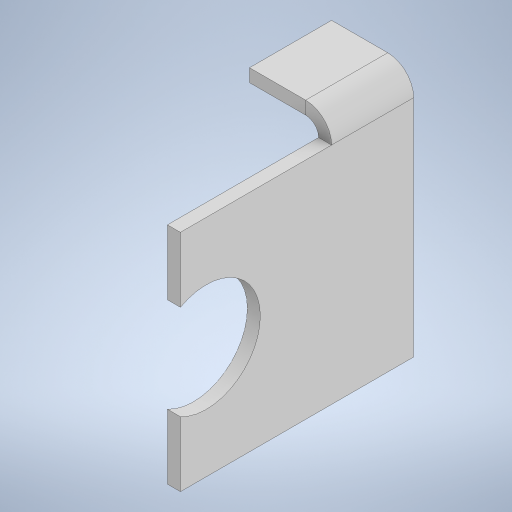
# Autodesk Inventor part: hipjoint_toleg_under_down_right
Saved by Autodesk Inventor 2024.1 (Build 281209000, 209)
## iProperties
Created: 2024-10-09
Part Number: hipjoint_toleg_under_down_right
Material: 一般
Document SubType Name: Sheet Metal
Designer: hibik
Density: 1 g/cm^3
Sheet Metal Rule: Default_mm
Appearance: 既定
Author: hibik
Autodesk Inventor part; units mm, degrees
ref_plane "YZ Plane" through (0, 0, 0) normal (1, 0, 0) x (0, 1, 0)
ref_plane "XZ Plane" through (0, 0, 0) normal (0, 1, 0) x (-1, 0, 0)
ref_plane "XY Plane" through (0, 0, 0) normal (0, 0, 1) x (1, 0, 0)
sketch "スケッチ2" plane through (0, 0, 0) normal (1, 0, 0) x (0, 1, 0)
  circle A0 centre (0, 0) radius 6.25
  line L0 (13, 0) -> (-13, 0) construction
  line L1 (-13, 0) -> (-13, -24)
  line L2 (-13, -24) -> (13, -24)
  line L3 (13, -24) -> (13, 0)
  line L4 (13, -24) -> (16, -24)
  line L5 (16, -24) -> (16, -14.5)
  line L6 (16, -14.5) -> (13, -14.5)
  line L7 (13, -14.5) -> (13, -24)
  line L8 (13, 0) -> (-13, 0)
  line L9 (-13, 0) -> (-13, 3)
  line L10 (-13, 3) -> (13, 3)
  line L11 (13, 3) -> (13, 0)
  point P0 (13, 0)
  point P1 (5.4829, 3)
  point P2 (-5.4829, 3)
  point P3 (-13, 0)
  dimension "d0" = 12.5
  dimension "d1" = 26
  dimension "d2" = 24
  dimension "d3" = 3
  dimension "d4" = 9.5
  dimension "d5" = 3
  measures "d0" diameter of A0
  measures "d1" distance of L2.end L1.end
  measures "d2" distance of L1.end L0.end
  measures "d3" distance of L6.end L5.end
  measures "d4" distance of L4.end L5.end
  measures "d5" distance of L8.end L9.end
extrude "プレート1" add sketch "スケッチ2" along normal blind 1.5 contours L8 L3 L2 L1 A0 | A0 L10 L11 L8 | L8 L9 L10 A0 | L6 L5 L4 L3
sketch "スケッチ3" plane through (1.5, 14.5, -24) normal (0, 1, 0) x (-1, 0, 0)
  line L0 (0, 9.5) -> (0, 0)
  line L1 (0, 0) -> (9.5, 0)
  line L2 (9.5, 0) -> (9.5, 9.5)
  line L3 (9.5, 9.5) -> (0, 9.5)
  constraints: 6 end point, 1 horizontal, 1 perpendicular, 1 vertical
edge flange "フランジ1" height 9.5 angle 90 thickness 1.5 bend radius 1.5 thickness toward (0, 1, 0) relief tear relief width 1.5 relief depth 0.75 edges at (0, 16, -19.25) wall of the first edge with corners at (1.5, 14.5, -14.5) (1.5, 14.5, -24) (-8, 14.5, -24) (-8, 14.5, -14.5)
bend "曲げ1"
corner "コーナー1"
equation "\"d6\" = Thickness"
equation "\"d7\" = BendReliefWidth"
equation "\"d8\" = BendReliefDepth"
equation "\"d9\" = MinimumRemnant"
equation "\"d10\" = TransitionRadius"
equation "\"d13\" = BendRadius"
equation "\"d14\" = CornerReliefSize"
equation "\"d15\" = GapSize"
equation "\"d16\" = JacobiRadiusSize"
equation "\"BendRadius\" = Thickness"
equation "\"BendReliefWidth\" = Thickness"
equation "\"BendReliefDepth\" = 0.5 * Thickness"
equation "\"CornerReliefSize\" = 4 * Thickness"
equation "\"MinimumRemnant\" = 2 * Thickness"
equation "\"TransitionRadius\" = BendRadius"
equation "\"JacobiRadiusSize\" = BendRadius"
equation "\"GapSize\" = Thickness"
equation "\"Thickness\" = 1.5"
